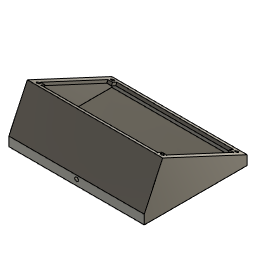
Body v1 (Autodesk Fusion 360 design; units mm, degrees)
Autodesk Fusion 360 part; units mm, degrees
sketch "Esquisse1" plane through (0, 0, 0) normal (0, 0, 1) x (1, 0, 0)
  line L0 (72.8914, -72.0117) -> (72.8914, -62.0006)
  line L1 (163.3271, -19.8297) -> (183.0909, -62.1224)
  line L2 (183.0691, -72.0117) -> (72.8914, -72.0117)
  line L3 (183.0909, -62.1224) -> (183.0691, -72.0117)
  line L4 (72.8914, -62.0006) -> (163.3271, -19.8297)
extrude "Extrusion1" add sketch "Esquisse1" along normal blind 145
move_body "Déplacer1" bodies 1 to x (1, 0, 0) y (0, 0, 1) z (0, -1, 0) at (0, 42.2239, 186.2473)
move_body "Déplacer2" bodies 1 to x (0, -1, 0) y (1, 0, 0) z (0, 0, 1) at (-118.9685, 114.7514, 0)
sketch "Esquisse2" plane through (-254.2414, -137.6605, 207.9585) normal (0, 0.422618, 0.906308) x (0, 0.906308, -0.422618)
  line L0 (122.7514, -122.1591) -> (122.7514, -136.1591)
  line L1 (130.4784, -50.1591) -> (144.4784, -50.1591)
  line L2 (122.7514, -112.1591) -> (108.7514, -112.1591)
  line L3 (108.7514, -88.1591) -> (108.7514, -74.1591)
  line L4 (108.7514, -112.1591) -> (108.7514, -98.1591)
  line L5 (130.4784, -64.1591) -> (130.4784, -50.1591)
  line L6 (152.2054, -159.6187) -> (152.2054, -145.6187)
  line L7 (152.2054, -145.6187) -> (166.2054, -145.6187)
  line L8 (130.4784, -98.1591) -> (144.4784, -98.1591)
  line L9 (166.2054, -159.6187) -> (152.2054, -159.6187)
  line L10 (130.4784, -145.6187) -> (144.4784, -145.6187)
  line L11 (130.4784, -88.1591) -> (130.4784, -74.1591)
  line L12 (130.4784, -122.1591) -> (144.4784, -122.1591)
  line L13 (122.7514, -88.1591) -> (108.7514, -88.1591)
  line L14 (144.4784, -88.1591) -> (130.4784, -88.1591)
  line L15 (130.4784, -112.1591) -> (130.4784, -98.1591)
  line L16 (166.2054, -145.6187) -> (166.2054, -159.6187)
  line L17 (122.7514, -136.1591) -> (108.7514, -136.1591)
  line L18 (144.4784, -159.6187) -> (130.4784, -159.6187)
  line L19 (108.7514, -136.1591) -> (108.7514, -122.1591)
  line L20 (108.7514, -145.6187) -> (122.7514, -145.6187)
  line L21 (122.7514, -145.6187) -> (122.7514, -159.6187)
  line L22 (108.7514, -122.1591) -> (122.7514, -122.1591)
  line L23 (108.7514, -159.6187) -> (108.7514, -145.6187)
  line L24 (108.7514, -74.1591) -> (122.7514, -74.1591)
  line L25 (108.7514, -50.1591) -> (122.7514, -50.1591)
  line L26 (130.4784, -159.6187) -> (130.4784, -145.6187)
  line L27 (130.4784, -136.1591) -> (130.4784, -122.1591)
  line L28 (166.2054, -122.1591) -> (166.2054, -136.1591)
  line L29 (144.4784, -50.1591) -> (144.4784, -64.1591)
  line L30 (144.4784, -74.1591) -> (144.4784, -88.1591)
  line L31 (108.7514, -98.1591) -> (122.7514, -98.1591)
  line L32 (122.7514, -50.1591) -> (122.7514, -64.1591)
  line L33 (144.4784, -145.6187) -> (144.4784, -159.6187)
  line L34 (144.4784, -112.1591) -> (130.4784, -112.1591)
  line L35 (122.7514, -159.6187) -> (108.7514, -159.6187)
  line L36 (122.7514, -98.1591) -> (122.7514, -112.1591)
  line L37 (130.4784, -74.1591) -> (144.4784, -74.1591)
  line L38 (144.4784, -64.1591) -> (130.4784, -64.1591)
  line L39 (108.7514, -64.1591) -> (108.7514, -50.1591)
  line L40 (122.7514, -64.1591) -> (108.7514, -64.1591)
  line L41 (122.7514, -74.1591) -> (122.7514, -88.1591)
  line L42 (166.2054, -112.1591) -> (152.2054, -112.1591)
  line L43 (98.3419, -32.524) -> (198.3419, -32.524)
  line L44 (152.2054, -98.1591) -> (166.2054, -98.1591)
  line L45 (173.9324, -98.4293) -> (187.9324, -98.4293)
  line L46 (173.9324, -136.4293) -> (173.9324, -122.4293)
  line L47 (173.9324, -64.4293) -> (173.9324, -50.4293)
  line L48 (166.2054, -74.1591) -> (166.2054, -88.1591)
  line L49 (166.2054, -88.1591) -> (152.2054, -88.1591)
  line L50 (166.2054, -64.1591) -> (152.2054, -64.1591)
  line L51 (187.9324, -64.4293) -> (173.9324, -64.4293)
  line L52 (173.9324, -145.8889) -> (187.9324, -145.8889)
  line L53 (187.9324, -98.4293) -> (187.9324, -112.4293)
  line L54 (152.2054, -112.1591) -> (152.2054, -98.1591)
  line L55 (144.4784, -122.1591) -> (144.4784, -136.1591)
  circle A0 centre (104.4919, -171.374) radius 1.8
  circle A1 centre (192.4919, -38.553) radius 1.8
  line L56 (166.2054, -98.1591) -> (166.2054, -112.1591)
  line L57 (187.9324, -136.4293) -> (173.9324, -136.4293)
  line L58 (187.9324, -88.4293) -> (173.9324, -88.4293)
  line L59 (144.4784, -98.1591) -> (144.4784, -112.1591)
  line L60 (187.9324, -145.8889) -> (187.9324, -159.8889)
  line L61 (173.9324, -50.4293) -> (187.9324, -50.4293)
  circle A2 centre (192.4919, -171.374) radius 1.8
  line L62 (173.9324, -74.4293) -> (187.9324, -74.4293)
  line L63 (187.9324, -159.8889) -> (173.9324, -159.8889)
  line L64 (166.2054, -50.1591) -> (166.2054, -64.1591)
  line L65 (173.9324, -112.4293) -> (173.9324, -98.4293)
  line L66 (152.2054, -88.1591) -> (152.2054, -74.1591)
  line L67 (173.9324, -122.4293) -> (187.9324, -122.4293)
  line L68 (187.9324, -74.4293) -> (187.9324, -88.4293)
  line L69 (198.3419, -177.524) -> (98.3419, -177.524)
  line L70 (98.3419, -177.524) -> (98.3419, -32.524)
  line L71 (152.2054, -64.1591) -> (152.2054, -50.1591)
  line L72 (152.2054, -122.1591) -> (166.2054, -122.1591)
  line L73 (152.2054, -50.1591) -> (166.2054, -50.1591)
  line L74 (187.9324, -112.4293) -> (173.9324, -112.4293)
  circle A3 centre (104.4919, -38.553) radius 1.8
  line L75 (198.3419, -32.524) -> (198.3419, -177.524)
  line L76 (173.9324, -159.8889) -> (173.9324, -145.8889)
  line L77 (166.2054, -136.1591) -> (152.2054, -136.1591)
  line L78 (173.9324, -88.4293) -> (173.9324, -74.4293)
  line L79 (152.2054, -74.1591) -> (166.2054, -74.1591)
  line L80 (187.9324, -122.4293) -> (187.9324, -136.4293)
  line L81 (187.9324, -50.4293) -> (187.9324, -64.4293)
  line L82 (152.2054, -136.1591) -> (152.2054, -122.1591)
  line L83 (144.4784, -136.1591) -> (130.4784, -136.1591)
  line L84 (17.5238, -15.2481) -> (31.5238, -15.2481)
  circle A4 centre (24.5238, -39.7717) radius 1.8
  line L85 (31.5238, -15.2481) -> (31.5238, -29.2481)
  line L86 (17.5238, -29.2481) -> (17.5238, -15.2481)
  line L87 (31.5238, -29.2481) -> (17.5238, -29.2481)
shell "Coque1" thickness 3 removed faces 1 at (-221.7446, -25.0184, 138.2631)
extrude "Extrusion2" cut sketch "Esquisse2" against normal blind 5 contours A0 | A1 | A2 | A3
sketch "Esquisse3" plane through (0, 55.0657, 118.0888) normal (0, 0.422618, 0.906308) x (-1, 0, 0)
  circle A0 centre (215.6883, 108.1579) radius 1.8
  circle A1 centre (215.6883, 20.1579) radius 1.8
  circle A2 centre (82.8673, 108.1579) radius 1.8
  circle A3 centre (82.8673, 20.1579) radius 1.8
  line L0 (76.7446, 114.3556) -> (76.7446, 14.5709)
  line L1 (76.7446, 14.5709) -> (221.7446, 14.5709)
  line L2 (221.7446, 14.5709) -> (221.7446, 114.3556)
  line L3 (221.7446, 114.3556) -> (76.7446, 114.3556)
  line L4 (221.7446, 114.3556) -> (211.7446, 114.3556)
  line L5 (211.7446, 114.3556) -> (211.7446, 104.3556)
  line L6 (211.7446, 104.3556) -> (221.7446, 104.3556)
  line L7 (221.7446, 104.3556) -> (221.7446, 114.3556)
  line L8 (76.7446, 114.3556) -> (86.7446, 114.3556)
  line L9 (86.7446, 114.3556) -> (86.7446, 104.3556)
  line L10 (86.7446, 104.3556) -> (76.7446, 104.3556)
  line L11 (76.7446, 104.3556) -> (76.7446, 114.3556)
  line L12 (76.7446, 14.5709) -> (86.7446, 14.5709)
  line L13 (86.7446, 14.5709) -> (86.7446, 24.5709)
  line L14 (86.7446, 24.5709) -> (76.7446, 24.5709)
  line L15 (76.7446, 24.5709) -> (76.7446, 14.5709)
  line L16 (221.7446, 14.5709) -> (211.7446, 14.5709)
  line L17 (211.7446, 14.5709) -> (211.7446, 24.5709)
  line L18 (211.7446, 24.5709) -> (221.7446, 24.5709)
  line L19 (221.7446, 24.5709) -> (221.7446, 14.5709)
  line L20 (81.7446, 104.3556) -> (216.7446, 104.3556)
  line L21 (216.7446, 104.3556) -> (216.7446, 24.5709)
  line L22 (216.7446, 24.5709) -> (81.7446, 24.5709)
  line L23 (81.7446, 24.5709) -> (81.7446, 104.3556)
  line L24 (86.7446, 109.3556) -> (211.7446, 109.3556)
  line L25 (211.7446, 109.3556) -> (211.7446, 104.3556)
  line L26 (211.7446, 104.3556) -> (86.7446, 104.3556)
  line L27 (86.7446, 104.3556) -> (86.7446, 109.3556)
  line L28 (86.7446, 24.5709) -> (211.7446, 24.5709)
  line L29 (211.7446, 24.5709) -> (211.7446, 19.5709)
  line L30 (211.7446, 19.5709) -> (86.7446, 19.5709)
  line L31 (86.7446, 19.5709) -> (86.7446, 24.5709)
  dimension "d6" = 10
  dimension "d7" = 10
  dimension "d8" = 10
  dimension "d9" = 10
  dimension "d10" = 10
  dimension "d11" = 10
  dimension "d12" = 10
  dimension "d13" = 10
  constraint horizontal L4
  constraint vertical L5
  constraint horizontal L6
  constraint vertical L7
  constraint coincident L2.end L3.start
  constraint horizontal L8
  constraint vertical L9
  constraint horizontal L10
  constraint vertical L11
  constraint coincident L0.start L3.end
  constraint horizontal L12
  constraint vertical L13
  constraint horizontal L14
  constraint vertical L15
  constraint coincident L0.end L1.start
  constraint horizontal L16
  constraint vertical L17
  constraint horizontal L18
  constraint vertical L19
  constraint coincident L1.end L2.start
  constraint horizontal L20
  constraint vertical L21
  constraint horizontal L22
  constraint vertical L23
  constraint midpoint L18 L21.end
  constraint midpoint L10 L20.start
  constraint horizontal L24
  constraint vertical L25
  constraint horizontal L26
  constraint vertical L27
  constraint midpoint L9 L24.start
  constraint horizontal L28
  constraint vertical L29
  constraint horizontal L30
  constraint vertical L31
  constraint midpoint L17 L29.end
  measures "d6" distance of L2.end L4.end
  measures "d7" distance of L2.end L6.end
  measures "d8" distance of L0.start L8.end
  measures "d9" distance of L0.start L10.end
  measures "d10" distance of L0.end L12.end
  measures "d11" distance of L0.end L14.end
  measures "d12" distance of L1.end L16.end
  measures "d13" distance of L1.end L18.end
extrude "Extrusion3" cut sketch "Esquisse3" against normal blind 5 contours L6 L10 L14 L18 L20 L21 L22 L23 L26 L28 | L5 L9 L20 L24 L25 L26 L27 | L13 L17 L22 L28 L29 L30 L31
sketch "Esquisse4" plane through (-221.7446, 0, 0) normal (-1, 0, 0) x (0, -1, 0)
  line L0 (-38.86, 122.3355) -> (47.1269, 162.4318)
  line L1 (47.1269, 162.4318) -> (65.338, 123.4617)
  line L2 (65.338, 123.4617) -> (65.3243, 117.2356)
  line L3 (65.3243, 117.2356) -> (-38.86, 117.2356)
  line L4 (-38.86, 117.2356) -> (-38.86, 122.3355)
  line L5 (-41.86, 124.2467) -> (-41.86, 114.2356)
  line L6 (-41.86, 114.2356) -> (68.3177, 114.2356)
  line L7 (68.3177, 114.2356) -> (68.3395, 124.125)
  line L8 (68.3395, 124.125) -> (48.5757, 166.4176)
  line L9 (48.5757, 166.4176) -> (-41.86, 124.2467)
extrude "Extrusion4" add sketch "Esquisse4" against normal blind 3 contours L0 L1 L2 L3 L4
hole "Perçage1" at (-149.2446, -65.3312, 120.3487) direction (0, -0.999998, -0.002198) diameter 4 depth 26 tip angle 118
